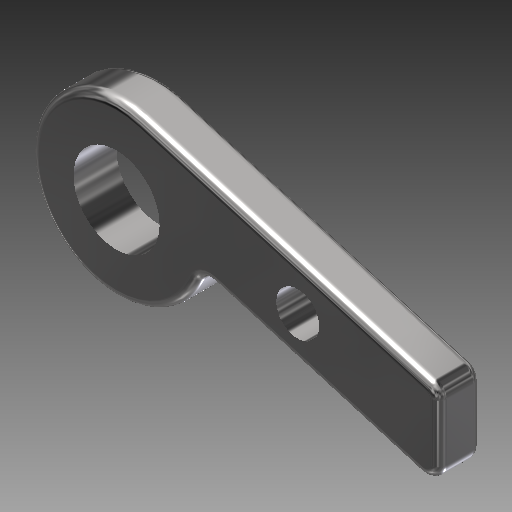
# Autodesk Inventor part: 403-05
Saved by Autodesk Inventor 2019 (Build 230136000, 136)
## iProperties
Company: Autodesk Inc.
Created: 2017-06-27
Part Number: 403-05
Material: Steel, Mild
Document SubType Name: Modeling
Designer: Autodesk Inc.
Mass: 0.518237 g
Surface Area: 1.55694 cm^2
Volume: 0.0660175 cm^3
Density: 7.85 g/cm^3
Appearance: Semi-Polished
Author: Inventor
Autodesk Inventor part; units mm, degrees
ref_plane "YZ Plane" through (0, 0, 0) normal (1, 0, 0) x (0, 1, 0)
ref_plane "XZ Plane" through (0, 0, 0) normal (0, 1, 0) x (-1, 0, 0)
ref_plane "XY Plane" through (0, 0, 0) normal (0, 0, 1) x (1, 0, 0)
sketch "Sketch1" plane through (0, 0, 0) normal (0, 0, 1) x (1, 0, 0)
  circle A0 centre (0, 0) radius 3
  line L0 (0.852, 2.8765) -> (11.2, -0.1887)
  line L1 (11.2, -0.1887) -> (11.2, -3.1887)
  line L2 (11.2, -3.1887) -> (2.9091, -0.7329)
  line L3 (0, 0) -> (-3, 0) construction
  dimension "d0" = 11.2
  dimension "d1" = 16.5
  dimension "d2" = 6
  dimension "d3" = 3
  constraints: 8 end point, 3 point on circle, 1 centre point, 1 coincident, 1 parallel, 1 perpendicular, 1 tangent, 1 vertical
  measures "d0" distance from line of L1 L3.start
  measures "d1" angle of L0 L3
  measures "d2" diameter of A0
  measures "d3" distance of L0.end L1.end
extrude "Extrusion1" add sketch "Sketch1" along normal blind 1.5
fillet "Fillet1" radius 0.5 3 edges at (2.9091, -0.7329, 0.75) (11.2, -3.1887, 0.75) (11.2, -0.1887, 0.75)
sketch "Sketch2" plane through (0, 0, 1.5) normal (0, 0, 1) x (1, 0, 0)
  line L0 (10.558, -2.9986) -> (3.3715, -0.8698) projected
  point P0 (0, 0)
  point P1 (6.3, -0.2772)
  dimension "d7" = 1.4
  dimension "d8" = 6.3
  measures "d7" distance from line of point (6.3, -0.277) L0
  measures "d8" horizontal distance of point (0, 0) point (6.3, -0.277)
hole "Hole1" at (6.3, -0.2772, 1.5) direction (0, 0, -1) diameter 1.5 end through all
hole "Hole2" at (0, 0, 1.5) direction (0, 0, -1) diameter 3 end through all
fillet "Fillet2" radius 0.3 14 edges at (11.1006, -0.2629, 1.5) (11.2, -1.5406, 1.5) (10.9992, -2.9198, 1.5) (6.9647, -1.9342, 1.5) (3.0149, -0.8976, 1.5) (-2.7097, -1.2874, 1.5) (5.847, 1.3969, 1.5) (10.9992, -2.9198, 0) (11.2, -1.5406, 0) (11.1006, -0.2629, 0) (5.847, 1.3969, 0) (-2.7097, -1.2874, 0) (3.0149, -0.8976, 0) (6.9647, -1.9342, 0)
body "Solid1"
